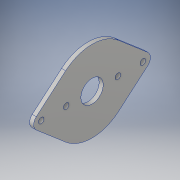
# Autodesk Inventor part: Motor Mount
Saved by Autodesk Inventor 2019.4 (Build 234330000, 330)
## iProperties
Created: 2020-01-16
Part Number: Motor Mount
Material: Aluminum 6061
Document SubType Name: Modeling
Designer: admin
Density: 2.7 g/cm^3
Appearance: Aluminum - Flat
Author: admin
Autodesk Inventor part; units mm, degrees
ref_plane "YZ Plane" through (0, 0, 0) normal (1, 0, 0) x (0, 1, 0)
ref_plane "XZ Plane" through (0, 0, 0) normal (0, 1, 0) x (-1, 0, 0)
ref_plane "XY Plane" through (0, 0, 0) normal (0, 0, 1) x (1, 0, 0)
sketch "Sketch1" plane through (0, 0, 0) normal (1, 0, 0) x (0, 1, 0)
  arc A0 (30.3974, 26) -> (-30.3974, 26) centre (0, 0) ccw construction
  circle A1 centre (0, 0) radius 25.4 construction
  circle A2 centre (0, 0) radius 11
  circle A3 centre (0, 50) radius 2.75
  circle A4 centre (0, -50) radius 2.75
  arc A5 (5.6995, -54.875) -> (-5.6995, -54.875) centre (0, -50) ccw construction
  arc A6 (-5.6995, 54.875) -> (5.6995, 54.875) centre (0, 50) ccw construction
  line L0 (0, 50) -> (0, 0) construction
  line L1 (0, 0) -> (0, -50) construction
  line L2 (5.6995, 54.875) -> (30.3974, 26)
  line L3 (30.3974, -26) -> (5.6995, -54.875)
  line L4 (-30.3974, -26) -> (-5.6995, -54.875)
  line L5 (-5.6995, 54.875) -> (-30.3974, 26)
  arc A7 (5.6995, 54.875) -> (-5.6995, 54.875) centre (0, 50) ccw
  arc A8 (-5.6995, -54.875) -> (5.6995, -54.875) centre (0, -50) ccw
  arc A9 (30.3974, -26) -> (30.3974, 26) centre (0, 0) ccw
  arc A10 (-30.3974, -26) -> (30.3974, -26) centre (0, 0) ccw construction
  arc A11 (-30.3974, 26) -> (-30.3974, -26) centre (0, 0) ccw
  circle A12 centre (0, 25.4) radius 2.75
  circle A13 centre (0, -25.4) radius 2.75
  line L6 (0, -25.4) -> (0, 25.4) construction
  dimension "d0" = 80
  dimension "d1" = 50.8
  dimension "d2" = 22
  dimension "d3" = 5.5
  dimension "d4" = 5.5
  dimension "d5" = 15
  dimension "d6" = 15
  dimension "d7" = 50
  dimension "d8" = 50
  dimension "d11" = 5.5
  dimension "d12" = 5.5
  constraints: 19 point on circle, 15 tangent, 14 centre point, 14 end point, 6 coincident, 2 vertical, 1 collinear, 1 midpoint
  measures "d0" diameter of A0
  measures "d1" diameter of A1
  measures "d2" diameter of A2
  measures "d3" diameter of A3
  measures "d4" diameter of A4
  measures "d5" diameter of A5
  measures "d6" diameter of A6
  measures "d7" distance of L0.start L0.end
  measures "d8" distance of L0.end L1.end
  measures "d11" diameter of A12
  measures "d12" diameter of A13
extrude "Extrusion1" add sketch "Sketch1" along normal blind 4
body "Solid1"
